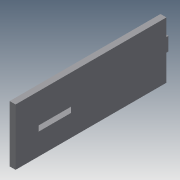
# Autodesk Inventor part: bt cover
Saved by Autodesk Inventor 2015 (Build 190159000, 159)
## iProperties
Created: 2017-05-24
Part Number: bt cover
Material: 일반
Document SubType Name: Modeling
Designer: gatew
Density: 1 g/cm^3
Appearance: 기본값
Author: gatew
Autodesk Inventor part; units mm, degrees
ref_plane "YZ Plane" through (0, 0, 0) normal (1, 0, 0) x (0, 1, 0)
ref_plane "XZ Plane" through (0, 0, 0) normal (0, 1, 0) x (-1, 0, 0)
ref_plane "XY Plane" through (0, 0, 0) normal (0, 0, 1) x (1, 0, 0)
sketch "스케치1" plane through (0, 0, 0) normal (1, 0, 0) x (0, 1, 0)
  line L0 (10.5, 28) -> (-10.5, 28)
  line L1 (-10.5, 28) -> (-10.5, -28)
  line L2 (-10.5, -28) -> (10.5, -28)
  line L3 (10.5, -28) -> (10.5, 28)
  line L4 (10.5, 28) -> (-10.5, -28) construction
  line L5 (-10.5, 28) -> (10.5, -28) construction
  point P0 (0, 0)
  dimension "d0" = 21
  dimension "d1" = 56
  constraints: 12 end point, 2 midpoint, 2 parallel, 1 horizontal, 1 perpendicular
  measures "d0" distance of L2.end L1.end
  measures "d1" distance of L1.end L0.end
extrude "돌출1" add sketch "스케치1" along normal blind 2.7
sketch "스케치2" plane through (0, -10.5, 28) normal (0, 0, 1) x (1, 0, 0)
  line L0 (0.31, 12) -> (2.01, 12)
  line L1 (2.01, 12) -> (2.01, 7)
  line L2 (2.01, 7) -> (0.31, 7)
  line L3 (0.31, 7) -> (0.31, 12)
  line L4 (0.31, 12) -> (2.01, 7) construction
  line L5 (2.01, 12) -> (0.31, 7) construction
  line L6 (-0.39, -0.5) -> (-0.39, 15)
  line L7 (-0.39, -0.5) -> (2.9, -0.5)
  line L8 (2.7, 0) -> (2.7, 21) projected
  line L9 (0, 0) -> (2.7, 0) projected
  point P0 (0, 10.5)
  point P1 (35, -7)
  point P2 (1.16, 9.5)
  dimension "d4" = 1.7
  dimension "d5" = 5
  dimension "d6" = 0.7
  dimension "d8" = 0.69
  dimension "d21" = 9.5
  constraints: 16 end point, 2 midpoint, 2 parallel, 1 horizontal, 1 perpendicular
  measures "d4" distance of L1.end L2.end
  measures "d5" distance of L0.end L1.end
  measures "d6" distance between parallel lines of L6 L3
  measures "d8" distance between parallel lines of L8 L1
  measures "d21" distance from line of L9 point (1.16, 9.5)
extrude "돌출2" add sketch "스케치2" along normal blind 1.95
chamfer "모따기1" distance 0.5 angle 45 8 edges at (0, -10.5, 0) (0, 0, 28) (0, 10.5, 0) (0, 0, -28) (2.01, -1, 29.95) (1.16, 1.5, 29.95) (0.31, -1, 29.95) (1.16, -3.5, 29.95)
sketch "스케치3" plane through (0, 0, 0) normal (0, 1, 0) x (-1, 0, 0)
  line L0 (-2.7, 28) -> (-2.7, -28) projected
  line L1 (-2.7, -7.4045) -> (-0.7, -3.9404)
  line L2 (-0.7, -3.9404) -> (-0.7, -19.4045)
  line L3 (-0.7, -19.4045) -> (-2.7, -19.4045)
  line L4 (-2.7, -19.4045) -> (-2.7, -7.4045)
  point P0 (0, 0)
  dimension "d18" = 12
  dimension "d19" = 30
  dimension "d20" = 2
  constraints: 8 end point, 2 point on line, 1 collinear, 1 perpendicular, 1 vertical
  measures "d18" distance of L3.end L1.start
  measures "d19" angle of L2 L1
  measures "d20" distance of L2.end L3.end
extrude "돌출4" cut sketch "스케치3" along normal mid plane 5
